# Autodesk Inventor part: C42_34
Saved by Autodesk Inventor 2015 SP1 (Build 190203100, 203)
## iProperties
Created: 2015-06-25
Part Number: C42_34
Material: Generic
Document SubType Name: Modeling
Designer: Patrick
Density: 1 g/cm^3
Appearance: C42_34, C42_34
Author: Patrick
Autodesk Inventor part; units mm, degrees
ref_plane "YZ Plane" through (0, 0, 0) normal (1, 0, 0) x (0, 1, 0)
ref_plane "XZ Plane" through (0, 0, 0) normal (0, 1, 0) x (-1, 0, 0)
ref_plane "XY Plane" through (0, 0, 0) normal (0, 0, 1) x (1, 0, 0)
sketch "C42_34, C42_34_208" plane through (0, 0, 0) normal (0, 0, 1) x (1, 0, 0)
  line L0 (-3.935, -2.665) -> (-3.935, 3.3)
  line L1 (-3.935, 3.3) -> (24.255, 3.3)
  line L2 (24.255, 3.3) -> (24.255, -2.665)
  line L3 (24.255, -2.665) -> (-3.935, -2.665)
  constraints: 8 end point
extrude "Extrusion1" add sketch "C42_34, C42_34_208" along normal blind 1
body "Solid1"
